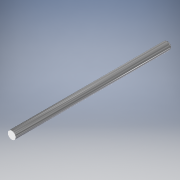
# Autodesk Inventor part: shaft
Saved by Autodesk Inventor 2019 (Build 230136000, 136)
## iProperties
Created: 2024-10-15
Part Number: shaft
Material: Aluminium 6061
Document SubType Name: Modeling
Designer: nic
Density: 2.7 g/cm^3
Appearance: Aluminium - flach
Author: nic
Autodesk Inventor part; units mm, degrees
ref_plane "YZ Plane" through (0, 0, 0) normal (1, 0, 0) x (0, 1, 0)
ref_plane "XZ Plane" through (0, 0, 0) normal (0, 1, 0) x (-1, 0, 0)
ref_plane "XY Plane" through (0, 0, 0) normal (0, 0, 1) x (1, 0, 0)
sketch "Skizze1" plane through (0, 0, 0) normal (0, 0, 1) x (1, 0, 0)
  circle A0 centre (0, 0) radius 1
  dimension "d0" = 2
  constraints: 1 centre point, 1 coincident
  measures "d0" diameter of A0
extrude "Extrusion1" add sketch "Skizze1" along normal blind 40
fillet "Rundung1" radius 0.5 1 edges at (-1, 0, 0)
